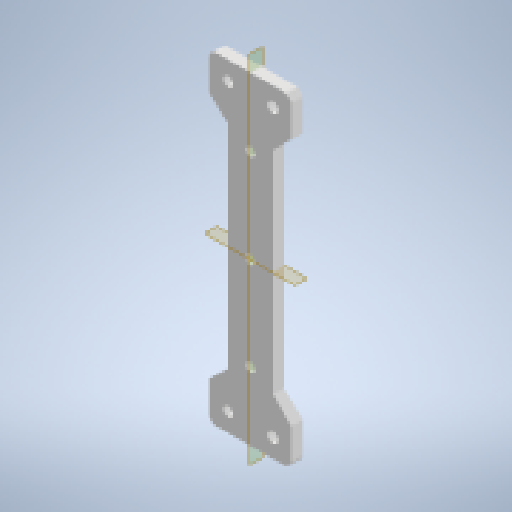
# Autodesk Inventor part: A-06
Saved by Autodesk Inventor 2023 (Build 270158000, 158)
## iProperties
Created: 2022-06-11
Part Number: A-06
Material: Generic
Document SubType Name: Modeling
Designer: kfcs7
Density: 1 g/cm^3
Appearance: Default
Author: kfcs7
Autodesk Inventor part; units mm, degrees
ref_plane "YZ Plane" through (0, 0, 0) normal (1, 0, 0) x (0, 1, 0)
ref_plane "XZ Plane" through (0, 0, 0) normal (0, 1, 0) x (-1, 0, 0)
ref_plane "XY Plane" through (0, 0, 0) normal (0, 0, 1) x (1, 0, 0)
sketch "Sketch1" plane through (0, 0, 0) normal (0, 0, 1) x (1, 0, 0)
  line L0 (12.5, 0) -> (18.7, 0) construction
  line L1 (12.5, 0) -> (12.5, -92) construction
  line L2 (12.5, -92) -> (18.7, -92) construction
  line L3 (18.7, -90.35) -> (18.7, -92) construction
  line L4 (18.7, -90.35) -> (19, -90.0495) construction
  line L5 (19, -90.0495) -> (19, -83.1505) construction
  line L6 (19, -83.1505) -> (18.7, -82.85) construction
  line L7 (18.7, -13.75) -> (18.7, -82.85) construction
  line L8 (18.7, -13.75) -> (19, -13.4495) construction
  line L9 (19, -13.4495) -> (19, -6.5505) construction
  line L10 (19, -6.5505) -> (18.7, -6.25) construction
  line L11 (18.7, 0) -> (18.7, -6.25) construction
  circle A0 centre (16, -86.6) radius 1.25 construction
  circle A1 centre (16, -10) radius 1.25 construction
  line L12 (0.5, 0) -> (6.7, 0) construction
  line L13 (0.5, 0) -> (0.5, -92) construction
  line L14 (0.5, -92) -> (6.7, -92) construction
  line L15 (6.7, -90.35) -> (6.7, -92) construction
  line L16 (6.7, -90.35) -> (7, -90.0495) construction
  line L17 (7, -90.0495) -> (7, -83.1505) construction
  line L18 (7, -83.1505) -> (6.7, -82.85) construction
  line L19 (6.7, -13.75) -> (6.7, -82.85) construction
  line L20 (6.7, -13.75) -> (7, -13.4495) construction
  line L21 (7, -13.4495) -> (7, -6.5505) construction
  line L22 (7, -6.5505) -> (6.7, -6.25) construction
  line L23 (6.7, 0) -> (6.7, -6.25) construction
  circle A2 centre (4, -86.6) radius 1.25 construction
  circle A3 centre (4, -10) radius 1.25 construction
  circle A4 centre (4, -86.6) radius 1.375
  circle A5 centre (16, -86.6) radius 1.375
  circle A6 centre (16, -10) radius 1.375
  circle A7 centre (4, -10) radius 1.375
  line L24 (4, -86.6) -> (4, -10) construction
  line L25 (4, -10) -> (16, -10) construction
  line L26 (16, -10) -> (16, -86.6) construction
  line L27 (16, -86.6) -> (4, -86.6) construction
  line L28 (-1, -5) -> (-1, -91.6)
  line L29 (-1, -91.6) -> (21, -91.6)
  line L30 (21, -91.6) -> (21, -5)
  line L31 (21, -5) -> (-1, -5)
  point P0 (0, 0)
  dimension "d0" = 2.75
  dimension "d1" = 2.75
  dimension "d2" = 2.75
  dimension "d3" = 2.75
  dimension "d4" = 5
  constraints: 16 end point, 5 coincident, 4 centre point, 4 parallel, 2 perpendicular, 1 vertical, 3 other
  measures "d0" diameter of A4
  measures "d1" diameter of A5
  measures "d2" diameter of A7
  measures "d3" diameter of A6
  measures "d4" distance between parallel lines of L24 L28
extrude "Extrusion1" add sketch "Sketch1" along normal blind 3
sketch "Sketch2" plane through (0, 0, 3) normal (0, 0, 1) x (1, 0, 0)
  line L0 (-1, -91.6) -> (21, -91.6) projected
  line L1 (21, -91.6) -> (21, -5) projected
  line L2 (21, -5) -> (-1, -5) projected
  line L3 (-1, -5) -> (-1, -91.6) projected
  circle A0 centre (4, -86.6) radius 1.375 projected
  circle A1 centre (16, -86.6) radius 1.375 projected
  circle A2 centre (16, -10) radius 1.375 projected
  circle A3 centre (4, -10) radius 1.375 projected
  line L4 (-1, -81.6) -> (4, -76.6)
  line L5 (4, -76.6) -> (4, -20)
  line L6 (4, -20) -> (-1, -15)
  point P0 (0, 0)
  dimension "d7" = 5
  dimension "d8" = 45
  dimension "d9" = 45
  dimension "d10" = 10
  dimension "d11" = 10
  constraints: 6 end point, 2 point on line, 1 vertical
  measures "d7" distance between parallel lines of L3 L5
  measures "d8" angle of L3 L4
  measures "d9" angle of L3 L6
  measures "d10" distance of L2.end L6.end
  measures "d11" distance of L0.start L4.start
extrude "Extrusion2" cut sketch "Sketch2" against normal through all contours L3 L6 L5 L4
ref_plane "Work Plane1" through (10, -91.6, 0) normal (-1, 0, 0) x (0, 0, 1)
mirror "Mirror1" about plane through (10, -91.6, 0) normal (-1, 0, 0) of "Extrusion2"
sketch "Sketch3" plane through (0, 0, 3) normal (0, 0, 1) x (1, 0, 0)
  line L0 (16, -20) -> (21, -15) projected
  line L1 (21, -15) -> (21, -5) projected
  line L2 (21, -5) -> (-1, -5) projected
  line L3 (-1, -5) -> (-1, -15) projected
  line L4 (-1, -15) -> (4, -20) projected
  line L5 (4, -20) -> (4, -76.6) projected
  line L6 (4, -76.6) -> (-1, -81.6) projected
  line L7 (-1, -81.6) -> (-1, -91.6) projected
  line L8 (-1, -91.6) -> (21, -91.6) projected
  line L9 (21, -91.6) -> (21, -81.6) projected
  line L10 (21, -81.6) -> (16, -76.6) projected
  line L11 (16, -76.6) -> (16, -20) projected
  circle A0 centre (4, -86.6) radius 1.375 projected
  circle A1 centre (16, -86.6) radius 1.375 projected
  circle A2 centre (16, -10) radius 1.375 projected
  circle A3 centre (4, -10) radius 1.375 projected
  circle A4 centre (10, -48.3) radius 1.25
  line L12 (10, -91.6) -> (10, -48.3)
  line L13 (10, -48.3) -> (4, -48.3)
  point P0 (0, 0)
  dimension "d14" = 2.5
  dimension "d15" = 43.3
  dimension "d16" = 86.6
  constraints: 4 end point, 2 midpoint, 1 centre point, 1 vertical
  measures "d14" diameter of A4
  measures "d15" distance of L12.start L12.end
  measures "d16" distance between parallel lines of L2 L8
extrude "Extrusion3" cut sketch "Sketch3" against normal through all contours L12 L13 A4 | A4 L13 L12
sketch "Sketch4" plane through (0, 0, 0) normal (0, 0, -1) x (-1, 0, 0)
  circle A0 centre (-10, -48.3) radius 1.25 projected
  line L0 (-10, -50.8981) -> (-12.25, -49.599)
  line L1 (-12.25, -49.599) -> (-12.25, -47.001)
  line L2 (-12.25, -47.001) -> (-10, -45.7019)
  line L3 (-10, -45.7019) -> (-7.75, -47.001)
  line L4 (-7.75, -47.001) -> (-7.75, -49.599)
  line L5 (-7.75, -49.599) -> (-10, -50.8981)
  line L6 (-4, -76.6) -> (-4, -20) projected
  point P0 (0, 0)
  dimension "d19" = 4.5
  constraints: 12 end point, 1 coincident, 1 parallel, 13 other
  measures "d19" distance between parallel lines of L4 L1
extrude "Extrusion4" cut sketch "Sketch4" against normal blind 2 contours A0 | L0 L1 L2 L3 L4 L5
pattern_linear "Rectangular Pattern1" count 3 spacing 25 along (0, -1, 0) of "Extrusion3", "Extrusion4" first direction both ways yes
ref_plane "Work Plane2" through (-1, -48.3, 0) normal (0, 1, 0) x (1, 0, 0)
fillet "Fillet1" radius 2 4 edges at (-1, -91.6, 1.5) (21, -91.6, 1.5) (-1, -5, 1.5) (21, -5, 1.5)
equation "\"d1\" = d0"
equation "\"d2\" = d0"
equation "\"d3\" = d0"
equation "\"d9\" = d8"
equation "\"d11\" = d10"
equation "\"d15\" = 0.5 * d16"
body "Solid1"
